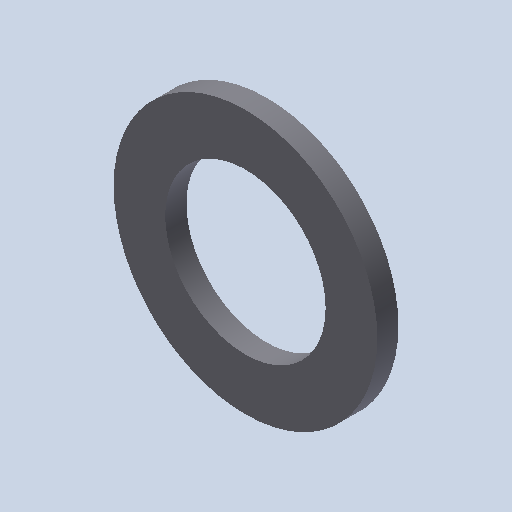
# Autodesk Inventor part: SPACER,SPROCKET,IDLER,ELEVATOR
Saved by Autodesk Inventor 2025.2 (Build 292293000, 293)
## iProperties
Category: _
Manager: _
ILogicPurgeVersion: 0.0.0.0
OnSaveVersion: 3.4.3.0
OnSaveAssembly: COREAutomationManager
Created: 2025-01-29
Part Number: SPACER,SPROCKET,IDLER,ELEVATOR
Checked By: 00
Engr Approved By: _
User Status: Work In Process
Material: Steel, MS
Description: STANDARD (mm)
Document SubType Name: Modeling
Mfg Approved By: John.Thibert
Designer: John.Thibert
Manufacturer: Standard
Standards Organization: Custom
Density: 7.86 g/cm^3
Appearance: Metal-Steel
CN_MASS: 0.0
CN_SERVICEABLE: _
FIRST_DESCRIPTION: _
SECOND_DESCRIPTION: _
THIRD_DESCRIPTION: _
ModelCat: Uncategorized
MaterialName: Steel, MS
Subject: _
Author: John.Thibert
Keywords: -
Revision Number: A
Autodesk Inventor part; units mm, degrees
ref_plane "YZ Plane" through (0, 0, 0) normal (1, 0, 0) x (0, 1, 0)
ref_plane "XZ Plane" through (0, 0, 0) normal (0, 1, 0) x (-1, 0, 0)
ref_plane "XY Plane" through (0, 0, 0) normal (0, 0, 1) x (1, 0, 0)
sketch "Sketch2" plane through (0, 0, 0) normal (0, 0, 1) x (1, 0, 0)
  circle A0 centre (0, 0) radius 4.826
  circle A1 centre (0, 0) radius 7.9375
  dimension "d0" = 9.652
  dimension "d1" = 15.875
  constraints: 2 centre point, 2 coincident
  measures "d0" diameter of A0
  measures "d1" diameter of A1
extrude "Extrusion1" add sketch "Sketch2" along normal mid plane 1.27
body "Solid1"
